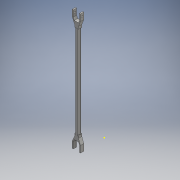
# Autodesk Inventor part: Rod v1
Saved by Autodesk Inventor 2016 (Build 200138000, 138)
## iProperties
Created: 2016-04-01
Part Number: Rod v1
Material: Generic
Document SubType Name: Modeling
Designer: Thetheos
Density: 1 g/cm^3
Appearance: Default
Author: Thetheos
Autodesk Inventor part; units mm, degrees
ref_plane "YZ Plane" through (0, 0, 0) normal (1, 0, 0) x (0, 1, 0)
ref_plane "XZ Plane" through (0, 0, 0) normal (0, 1, 0) x (-1, 0, 0)
ref_plane "XY Plane" through (0, 0, 0) normal (0, 0, 1) x (1, 0, 0)
sketch "Sketch1" plane through (0, 0, 0) normal (0, 0, 1) x (1, 0, 0)
  line L0 (9.75, 13) -> (7.875, 9.7524)
  line L1 (7.875, 9.7524) -> (4.125, 9.7524)
  line L2 (4.125, 9.7524) -> (2.25, 13)
  line L3 (2.25, 13) -> (4.125, 16.2476)
  line L4 (4.125, 16.2476) -> (7.875, 16.2476)
  line L5 (7.875, 16.2476) -> (9.75, 13)
  point P0 (0, 0)
  point P1 (6, 13)
  dimension "d0" = 7.5
  constraints: 12 end point, 13 other
  measures "d0" distance of L0.start L2.end
extrude "Extrusion1" add sketch "Sketch1" along normal blind 180
sketch "Sketch2" plane through (4.125, 16.2476, 0) normal (0, 1, 0) x (1, 0, 0)
  line L0 (3.75, -180) -> (5.625, -180) projected
  line L1 (3.75, -180) -> (0, -180) projected
  line L2 (0, -180) -> (-6.6597, -195.0128)
  line L3 (-1.875, 0) -> (-1.875, -180) projected
  line L4 (-6.6597, -207.8247) -> (-6.6597, -195.0128)
  line L5 (3.75, -180) -> (1.875, -180)
  line L6 (9.3403, -207.8668) -> (9.3403, -194.8539)
  line L7 (9.3403, -194.8539) -> (3.75, -180)
  line L8 (9.3403, -207.8668) -> (7.3403, -207.8668)
  line L9 (7.3403, -207.8668) -> (7.3403, -195.2178)
  line L10 (-6.6597, -207.8247) -> (-4.6597, -207.8247)
  line L11 (-4.6597, -207.8247) -> (-4.6597, -195.4364)
  line L12 (2.1735, -180.0436) -> (2.158, -180)
  line L13 (1.875, -191) -> (5.7529, -191)
  line L14 (-2.6917, -191) -> (1.875, -191)
  line L15 (-4.6597, -195.4364) -> (-2.6917, -191)
  line L16 (5.7529, -191) -> (7.3403, -195.2178)
  line L17 (1.875, -180) -> (1.875, -207.8247)
  point P0 (-4.125, 0)
  dimension "d12" = 2
  dimension "d13" = 2
  dimension "d16" = 27.8247
  dimension "d17" = 11
  dimension "d21" = 12
  dimension "d31" = 2
  dimension "d32" = 2
  constraints: 30 end point, 3 parallel, 3 vertical, 2 horizontal, 2 perpendicular, 2 point on line, 1 collinear, 1 midpoint
  measures "d12" distance of L6.start L8.end
  measures "d13" distance of L4.start L10.end
  measures "d16" distance between parallel lines of L10 L1
  measures "d17" distance of L5.end L13.start
  measures "d21" distance between parallel lines of L9 L11
  measures "d31" distance between parallel lines of L2 L15
  measures "d32" distance between parallel lines of L7 L16
extrude "Extrusion2" add sketch "Sketch2" against normal blind 6.5
sketch "Sketch3" plane through (-2.5347, 9.7476, 195.0128) normal (-0.9141, 0, -0.4055) x (-0.4055, 0, 0.9141)
  point P0 (-179.2885, -9.7476)
sketch "Sketch5" plane through (4.125, 16.2476, 0) normal (0, 1, 0) x (1, 0, 0)
  line L0 (-1.875, -180) -> (0, -180) projected
  line L1 (-1.875, -180) -> (-1.875, -184.2268)
  line L2 (0, -180) -> (-6.6597, -195.0128) projected
  line L3 (3.75, -180) -> (5.625, -180) projected
  line L4 (5.625, -180) -> (5.625, -184.982)
  line L5 (9.3403, -194.8539) -> (3.75, -180) projected
  point P0 (-4.125, 0)
  constraints: 4 end point, 2 perpendicular, 2 point on line, 1 parallel, 1 vertical
extrude "Extrusion3" add sketch "Sketch5" against normal blind 6.5
sketch "Sketch6" plane through (13.4653, 16.2476, 207.8668) normal (1, 0, 0) x (0, 0, -1)
  line L0 (0, 0) -> (0, -3.25)
  line L1 (0, 0) -> (0, -6.5) projected
  line L2 (0, -3.25) -> (6, -3.25)
  circle A0 centre (6, -3.25) radius 1.5
  point P0 (207.8668, -16.2476)
  dimension "d27" = 6
  dimension "d28" = 3
  constraints: 4 end point, 1 centre point, 1 coincident, 1 midpoint
  measures "d27" distance of L0.end L2.end
  measures "d28" diameter of A0
extrude "Extrusion4" cut sketch "Sketch6" against normal through all
sketch "Sketch7" plane through (4.125, 9.7524, 0) normal (0, -1, 0) x (1, 0, 0)
  line L0 (0, 0) -> (-6.6005, -15.1699)
  line L1 (-6.6005, -27.9818) -> (-6.6005, -15.1699)
  line L2 (9.3995, -28.0239) -> (9.3995, -15.011)
  line L3 (9.3995, -15.011) -> (3.75, 0)
  line L4 (9.3995, -28.0239) -> (7.3995, -28.0239)
  line L5 (7.3995, -28.0239) -> (7.3995, -15.3749)
  line L6 (-6.6005, -27.9818) -> (-4.6005, -27.9818)
  line L7 (-4.6005, -27.9818) -> (-4.6005, -15.5861)
  line L8 (1.9054, -10.9999) -> (5.7124, -10.8924)
  line L9 (-2.6612, -11.129) -> (1.9054, -10.9999)
  line L10 (-4.6005, -15.5861) -> (-2.6612, -11.129)
  line L11 (5.7124, -10.8924) -> (7.3995, -15.3749)
  line L12 (1.942, 0) -> (1.942, -27.8247)
  line L13 (5.625, 0) -> (3.75, 0) projected
  line L14 (0, 0) -> (3.75, 0) projected
  line L15 (3.75, 0) -> (0, 0)
  line L16 (3.75, 0) -> (0, 0) projected
  point P0 (-4.125, 0)
  dimension "d34" = 2
  dimension "d35" = 2
  dimension "d36" = 11
  dimension "d37" = 12
  dimension "d38" = 2
  dimension "d39" = 2
  constraints: 28 end point, 3 horizontal, 3 vertical, 2 parallel, 2 perpendicular, 2 point on line, 1 collinear
  measures "d34" distance of L2.start L4.end
  measures "d35" distance of L1.start L7.start
  measures "d36" distance of L12.start L9.end
  measures "d37" distance between parallel lines of L5 L7
  measures "d38" distance between parallel lines of L0 L10
  measures "d39" distance between parallel lines of L3 L11
extrude "Extrusion5" add sketch "Sketch7" against normal blind 6.5
sketch "Sketch8" plane through (1.4333, 16.2476, 191) normal (0, 1, 0) x (1, 0, 0)
  line L0 (8.3167, 191) -> (6.4417, 191) projected
  line L1 (8.3167, 191) -> (8.3167, 195.982)
  line L2 (12.0911, 206.011) -> (6.4417, 191) projected
  line L3 (2.6917, 191) -> (0.8167, 191) projected
  line L4 (0.8167, 191) -> (0.8167, 195.3093)
  line L5 (-3.9089, 206.1699) -> (2.6917, 191) projected
  point P0 (-1.4333, 191)
  constraints: 4 end point, 2 perpendicular, 2 point on line, 2 vertical, 1 parallel
extrude "Extrusion6" add sketch "Sketch8" against normal blind 6.5
body "Solid1"
